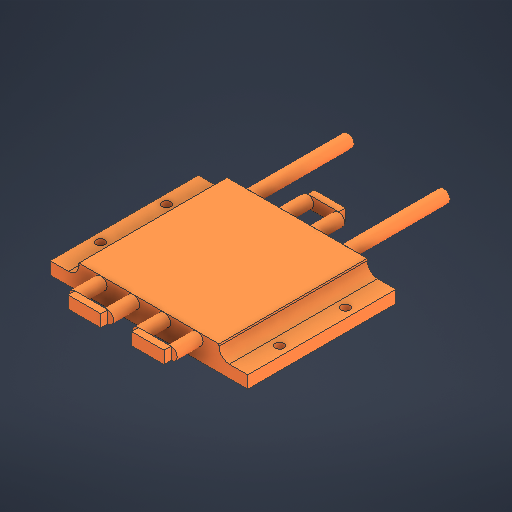
# Autodesk Inventor part: cooling plate
Saved by Autodesk Inventor 2025.2 (Build 292293000, 293)
## iProperties
Created: 2024-12-04
Part Number: cooling plate
Material: Generic
Document SubType Name: Modeling
Designer: cbast
Density: 1 g/cm^3
Appearance: Default
Author: cbast
Autodesk Inventor part; units mm, degrees
ref_plane "YZ Plane" through (0, 0, 0) normal (1, 0, 0) x (0, 1, 0)
ref_plane "XZ Plane" through (0, 0, 0) normal (0, 1, 0) x (-1, 0, 0)
ref_plane "XY Plane" through (0, 0, 0) normal (0, 0, 1) x (1, 0, 0)
sketch "Sketch1" plane through (0, 0, 0) normal (0, 1, 0) x (-1, 0, 0)
  line L0 (-76.2, 57.15) -> (76.2, 57.15)
  line L1 (76.2, 57.15) -> (76.2, -57.15)
  line L2 (76.2, -57.15) -> (-76.2, -57.15)
  line L3 (-76.2, -57.15) -> (-76.2, 57.15)
  line L4 (-76.2, 57.15) -> (76.2, -57.15) construction
  line L5 (76.2, 57.15) -> (-76.2, -57.15) construction
  point P0 (0, 0)
  dimension "d0" = 152.4
  dimension "d1" = 114.3
  constraints: 12 end point, 2 midpoint, 2 parallel, 1 horizontal, 1 perpendicular
  measures "d0" distance of L1.end L2.end
  measures "d1" distance of L0.end L1.end
extrude "Extrusion1" add sketch "Sketch1" along normal blind 9.55
sketch "Sketch2" plane through (0, 9.55, 0) normal (0, 1, 0) x (1, 0, 0)
  line L0 (54, -57.15) -> (-54, -57.15)
  line L1 (-54, -57.15) -> (-54, 57.15)
  line L2 (-54, 57.15) -> (54, 57.15)
  line L3 (54, 57.15) -> (54, -57.15)
  line L4 (54, -57.15) -> (-54, 57.15) construction
  line L5 (-54, -57.15) -> (54, 57.15) construction
  point P0 (0, 0)
  dimension "d4" = 108
  dimension "d5" = 114.3
  constraints: 12 end point, 2 midpoint, 2 parallel, 1 horizontal, 1 perpendicular
  measures "d4" distance of L1.end L2.end
  measures "d5" distance of L0.end L1.end
extrude "Extrusion2" add sketch "Sketch2" along normal blind 9.55
fillet "Fillet1" radius 8 1 edges at (-54, 9.55, 0)
fillet "Fillet2" radius 8 1 edges at (54, 9.55, 0)
sketch "Sketch3" plane through (-76.2, 0, 57.15) normal (0, 0, 1) x (1, 0, 0)
  line L0 (0, 0) -> (0, 9.55) construction
  line L1 (0, 9.55) -> (0, 14.325) construction
  line L2 (0, 14.325) -> (152.4, 14.325) construction
  circle A0 centre (39.2, 14.325) radius 4.7625
  circle A1 centre (64.2, 14.325) radius 4.7625
  circle A2 centre (88.2, 14.325) radius 4.7625
  circle A3 centre (113.2, 14.325) radius 4.7625
  arc A4 (130.2, 17.55) -> (138.2, 9.55) centre (138.2, 17.55) ccw projected
  arc A5 (14.2, 9.55) -> (22.2, 17.55) centre (14.2, 17.55) ccw projected
  point P0 (76.2, 0)
  dimension "d10" = 9.55
  dimension "d11" = 4.775
  dimension "d12" = 152.4
  dimension "d13" = 9.525
  dimension "d14" = 9.525
  dimension "d15" = 9.525
  dimension "d16" = 9.525
  dimension "d17" = 25
  dimension "d18" = 25
  dimension "d19" = 25
  dimension "d20" = 25
  constraints: 6 end point, 5 point on line, 4 centre point, 1 perpendicular, 1 vertical
  measures "d10" distance of L0.start L0.end
  measures "d11" distance of L0.end L1.end
  measures "d12" distance of L1.end L2.end
  measures "d13" diameter of A0
  measures "d14" diameter of A1
  measures "d15" diameter of A2
  measures "d16" diameter of A3
  measures "d17" horizontal distance of A4.centre A3.centre
  measures "d18" distance of A3.centre A2.centre
  measures "d19" horizontal distance of A5.centre A0.centre
  measures "d20" distance of A1.centre A0.centre
extrude "Extrusion3" add sketch "Sketch3" along normal blind 20
sketch "Sketch4" plane through (-37, 14.325, 77.15) normal (0, 0, 1) x (1, 0, 0)
  line L0 (-0.0011, 4.7559) -> (25.2383, 4.7559)
  line L1 (25.2383, 4.7559) -> (25.2383, -4.6618)
  line L2 (25.2383, -4.6618) -> (-0.0011, -4.6618)
  line L3 (-0.0011, -4.6618) -> (-0.0011, 4.7559)
  point P0 (37, -14.325)
  constraints: 8 end point, 2 parallel, 1 horizontal, 1 perpendicular
extrude "Extrusion4" add sketch "Sketch4" along normal blind 5.4
sketch "Sketch5" plane through (12, 14.325, 77.15) normal (0, 0, 1) x (1, 0, 0)
  line L0 (0.0017, 4.7559) -> (25.0231, 4.7559)
  line L1 (25.0231, 4.7559) -> (25.0231, -4.7498)
  line L2 (25.0231, -4.7498) -> (0.0017, -4.7498)
  line L3 (0.0017, -4.7498) -> (0.0017, 4.7559)
  point P0 (-12, -14.325)
  constraints: 8 end point, 2 parallel, 1 horizontal, 1 perpendicular
extrude "Extrusion5" add sketch "Sketch5" along normal blind 5.4
sketch "Sketch6" plane through (76.2, 0, -57.15) normal (0, 0, -1) x (-1, 0, 0)
  circle A0 centre (39.2, 14.325) radius 4.7625 projected
  circle A1 centre (113.2, 14.325) radius 4.7625 projected
  circle A2 centre (39.2, 14.325) radius 4.7625
  circle A3 centre (113.2, 14.325) radius 4.7625
  point P0 (76.2, 0)
  constraints: 2 centre point, 2 coincident, 2 concentric
extrude "Extrusion6" add sketch "Sketch6" along normal blind 76.2
sketch "Sketch7" plane through (76.2, 0, -57.15) normal (0, 0, -1) x (-1, 0, 0)
  circle A0 centre (64.2, 14.325) radius 4.7625 projected
  circle A1 centre (88.2, 14.325) radius 4.7625 projected
  circle A2 centre (64.2, 14.325) radius 4.7625
  circle A3 centre (88.2, 14.325) radius 4.7625
  point P0 (76.2, 0)
  constraints: 2 centre point, 2 coincident, 2 concentric
extrude "Extrusion7" add sketch "Sketch7" along normal blind 20
sketch "Sketch8" plane through (12, 14.325, -77.15) normal (0, 0, -1) x (-1, 0, 0)
  line L0 (-0.0002, 4.7633) -> (24.1286, 4.7633)
  line L1 (24.1286, 4.7633) -> (24.1286, -4.7128)
  line L2 (24.1286, -4.7128) -> (-0.0002, -4.7128)
  line L3 (-0.0002, -4.7128) -> (-0.0002, 4.7633)
  point P0 (12, -14.325)
  constraints: 8 end point, 2 parallel, 1 horizontal, 1 perpendicular
extrude "Extrusion8" add sketch "Sketch8" along normal blind 5.4
sketch "Sketch9" plane through (0, 9.55, 0) normal (0, 1, 0) x (1, 0, 0)
  line L0 (-76.2, 57.15) -> (-76.2, -57.15) construction
  line L1 (-76.2, -57.15) -> (-62, -57.15) construction
  line L2 (-62, 57.15) -> (-62, -57.15) construction
  line L3 (-62, 57.15) -> (-76.2, 57.15) construction
  line L4 (76.2, 57.15) -> (62, 57.15) construction
  line L5 (76.2, -57.15) -> (76.2, 57.15) construction
  line L6 (62, -57.15) -> (62, 57.15) construction
  line L7 (62, -57.15) -> (76.2, -57.15) construction
  line L8 (-76.2, -57.15) -> (-62, -57.15) construction
  line L9 (-69.1, 0) -> (-69.1, -25.4) construction
  line L10 (-69.1, 0) -> (-69.1, 25.4) construction
  circle A0 centre (-69.1, 25.4) radius 3.365
  circle A1 centre (-69.1, -25.4) radius 3.365
  point P0 (0, 0)
  dimension "d36" = 25.4
  dimension "d37" = 25.4
  dimension "d38" = 6.73
  dimension "d39" = 6.73
  constraints: 6 end point, 2 centre point, 2 coincident, 1 collinear, 1 parallel
  measures "d36" distance of L9.start L9.end
  measures "d37" distance of L9.start L10.end
  measures "d38" diameter of A0
  measures "d39" diameter of A1
extrude "Extrusion9" cut sketch "Sketch9" against normal blind 10
ref_plane "Work Plane1" through (-0.0642, 19.0883, -82.55) normal (-1, 0, 0) x (0, 0, 1)
mirror "Mirror1" about plane through (-0.0642, 19.0883, -82.55) normal (-1, 0, 0) of "Extrusion9"
body "Solid1"
